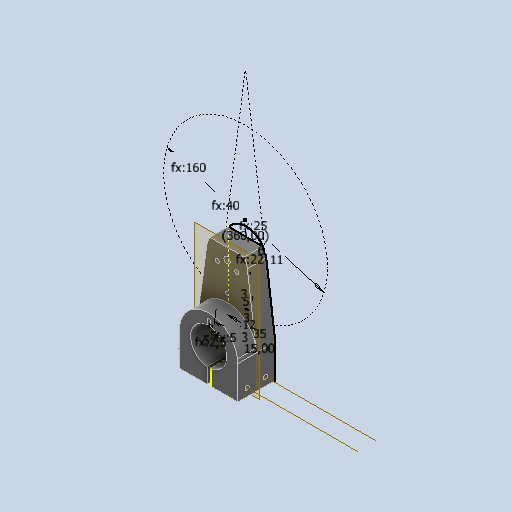
# Autodesk Inventor part: GC_Motor_Aussenscheibe
Saved by Autodesk Inventor 2022 (Build 260153000, 153)
## iProperties
Created: 2022-08-03
Part Number: GC_Motor_Aussenscheibe
Material: PBT-Kunststoff
Document SubType Name: Modeling
Designer: alexw
Mass: 147.379 g
Surface Area: 260.819 cm^2
Volume: 112.503 cm^3
Density: 1.31 g/cm^3
Appearance: Glatt - Schwarz
Author: alexw
Autodesk Inventor part; units mm, degrees
ref_plane "YZ Plane" through (0, 0, 0) normal (1, 0, 0) x (0, 1, 0)
ref_plane "XZ Plane" through (0, 0, 0) normal (0, 1, 0) x (-1, 0, 0)
ref_plane "XY Plane" through (0, 0, 0) normal (0, 0, 1) x (1, 0, 0)
sketch "Skizze1" plane through (0, 0, 0) normal (0, 0, 1) x (1, 0, 0)
  circle A0 centre (0, 0) radius 20 construction
  line L0 (-19.8289, 2.6105) -> (-28.5983, -64)
  line L1 (19.8289, 2.6105) -> (28.5983, -64)
  circle A1 centre (0, 0) radius 11 construction
  line L2 (0, 0) -> (0, 20) construction
  line L3 (0, 0) -> (0, -96.5) construction
  circle A2 centre (0, -64) radius 17.5
  line L4 (-19.8289, 2.6105) -> (0, 153.226) construction
  line L5 (19.8289, 2.6105) -> (0, 153.226) construction
  circle A3 centre (0, 25) radius 80 construction
  circle A4 centre (0, -64) radius 6 construction
  arc A5 (19.8289, 2.6105) -> (-19.8289, 2.6105) centre (0, 0) ccw
  line L6 (28.5983, -64) -> (28.5983, -96.5)
  line L7 (28.5983, -96.5) -> (-28.5983, -96.5)
  line L8 (-28.5983, -96.5) -> (-28.5983, -64)
  line L9 (0, -64) -> (-28.5983, -64) construction
  line L10 (0, -89) -> (-28.5983, -89) construction
  line L11 (0, -86.5) -> (-28.5983, -86.5) construction
  line L12 (0, -91.5) -> (-28.5983, -91.5) construction
  line L13 (1.5, -64) -> (-1.5, -64)
  line L14 (-1.5, -64) -> (-1.5, -96.5)
  line L15 (-1.5, -96.5) -> (1.5, -96.5)
  line L16 (1.5, -96.5) -> (1.5, -64)
  line L17 (-16.7033, 11) -> (16.7033, 11)
  circle A6 centre (0, 0) radius 3
  line L18 (-1.5, -46.5644) -> (-1.5, -41.5644)
  arc A7 (1.5, -41.5644) -> (-1.5, -41.5644) centre (0, -41.5644) ccw
  line L19 (1.5, -41.5644) -> (1.5, -46.5644)
  line L20 (1.5, -46.5644) -> (-1.5, -46.5644)
  point P0 (0, 11)
  point P1 (-9.5263, -5.5)
  point P2 (9.5263, -5.5)
  point P3 (0, -55)
  point P4 (0, -58)
  point P5 (0, -46.5)
  point P6 (0, -81.5)
  point P7 (-1.5, -81.4356)
  point P8 (1.5, -81.4356)
  point P9 (0, -46.5644)
  dimension "d9" = 22
  dimension "d54" = 160
  dimension "d56" = 12
  dimension "d2" = 360
  dimension "d10" = 40
  dimension "d47" = 25
  dimension "d51" = 3
  dimension "d52" = 15
  dimension "d55" = 35
  dimension "d61" = 5
  dimension "d62" = 2.5
  dimension "d63" = 5
  dimension "d65" = 3
  dimension "d66" = 5
  dimension "d81" = 11
  dimension "d82" = 6
  dimension "d85" = 3
  dimension "d86" = 5
  constraints: 40 end point, 13 point on circle, 7 perpendicular, 6 point on line, 6 tangent, 5 centre point, 5 coincident, 3 collinear, 3 horizontal, 3 midpoint, 3 parallel, 3 vertical, 3 vertical alignment, 1 equal length, 22 other
  measures "d10" diameter of A0
  measures "d47" distance of point (0, 25) point (0, 0)
  measures "d51" distance of point (0, -58) point (0, -55)
  measures "d52" angle of L1 L0
  measures "d55" diameter of A2
  measures "d61" distance between parallel lines of L11 L12
  measures "d62" distance between parallel lines of L12 L10
  measures "d63" distance between parallel lines of L12 L7
  measures "d65" distance between parallel lines of L14 L16
  measures "d66" distance from line of L11 A2.end
  measures "d81" distance from line of L17 point (0, 0)
  measures "d82" diameter of A6
  measures "d85" distance between parallel lines of L18 L19
  measures "d86" distance from line of A7.centre L20
extrude "Extrusion1" add sketch "Skizze1" along normal blind 18 contours A5 L17 L1 L6 L7 L16 A2 L19 A7 L18 L14 L8 L0
hole "Bohrung1" at (-9.5263, -5.5, 0) at (9.5263, -5.5, 0) direction (0, 0, 1) diameter 4 end through all
sketch "Skizze4" plane through (0, 0, 18) normal (0, 0, 1) x (1, 0, 0)
  circle A0 centre (0, -64) radius 28.3537
  line L0 (28.5983, -64) -> (19.8289, 2.6105) projected
  line L1 (-28.5983, -64) -> (-28.5983, -96.5) projected
  line L2 (-19.8289, 2.6105) -> (-28.5983, -64) projected
  line L3 (28.5983, -96.5) -> (28.5983, -64) projected
  line L4 (1.5, -96.5) -> (28.5983, -96.5) projected
  line L5 (-28.5983, -96.5) -> (-1.5, -96.5) projected
  line L6 (-1.5, -96.5) -> (-1.5, -81.4356) projected
  arc A1 (1.5, -81.4356) -> (-1.5, -81.4356) centre (0, -64) ccw projected
  line L7 (1.5, -81.4356) -> (1.5, -96.5) projected
  line L8 (1.5, -96.5) -> (1.5, -81.4356)
  line L9 (-1.5, -46.5644) -> (-1.5, -41.5644) projected
  arc A2 (1.5, -41.5644) -> (-1.5, -41.5644) centre (0, -41.5644) ccw projected
  line L10 (1.5, -41.5644) -> (1.5, -46.5644) projected
  line L11 (1.5, -46.5644) -> (-1.5, -46.5644) projected
  point P0 (0, 0)
  point P1 (28.1111, -60.2991)
  point P2 (-28.1111, -60.2991)
  constraints: 2 end point, 1 centre point, 1 coincident, 1 tangent, 1 vertical
extrude "Extrusion2" add sketch "Skizze4" along normal blind 18 contours A0 L7 A1 L10 A2 L9 L6 | A0 L0 L3 L4 L7 | A0 L6 L5 L1 L2
ref_plane "Arbeitsebene1" through (0, 0, 18) normal (0, 0, 1) x (1, 0, 0)
sketch "Skizze2" plane through (1.5, -96.5, 0) normal (-1, 0, 0) x (0, 0, 1)
  line L0 (0, 15.0644) -> (0, 0) construction
  line L1 (0, 0) -> (36, 0) construction
  line L2 (0, 15.0644) -> (36, 15.0644) construction
  line L3 (0, 0) -> (18, 0) construction
  line L4 (0, 15.0644) -> (18, 0) construction
  line L5 (18, 15.0644) -> (0, 0) construction
  line L6 (36, 15.0644) -> (36, 0) projected
  line L7 (18, 129) -> (18, -21.5) construction
  point P0 (0, 96.5)
  point P1 (9, 7.5322)
  point P2 (27, 7.5322)
  constraints: 4 end point, 2 midpoint, 1 symmetric about line
hole "Bohrung3" at (1.5, -88.9678, 9) at (1.5, -88.9678, 27) direction (1, 0, 0) diameter 4.134 end through all thread size "M5x0.8" class "6H" standard "ISO Metric profile"
sketch "Skizze3" plane through (-28.5983, -96.5, 0) normal (-1, 0, 0) x (0, 0, 1)
  point P0 (0, 96.5)
  point P1 (9, 7.5322)
  point P2 (27, 7.5322)
hole "Bohrung4" at (-28.5983, -88.9678, 9) at (-28.5983, -88.9678, 27) direction (1, 0, 0) diameter 5.5 depth 27.0983 tip angle 118 counterbore diameter 10 counterbore depth 5.5 clearance for "Inbusschraube DIN EN ISO 4762" size "M5" standard "DIN"
sketch "Skizze5" plane through (1.5, -96.5, 0) normal (0, -1, 0) x (1, 0, 0)
  line L0 (38.5377, 27) -> (-41.5377, 27) construction
  line L1 (38.5377, 9) -> (-41.5377, 9) construction
  line L2 (-41.5377, 18) -> (38.5377, 18) construction
  line L3 (-3, 36) -> (0, 36) construction
  line L4 (-1.5, 36) -> (-1.5, 0) construction
  point P0 (13.5, 18)
  point P1 (-16.5, 18)
  dimension "d87" = 15
  dimension "d88" = 30
  constraints: 2 end point, 2 point on line, 1 midpoint, 1 vertical
  measures "d87" distance from line of point (13.5, 18) L4
  measures "d88" distance of point (13.5, 18) point (-16.5, 18)
hole "Bohrung5" at (15, -96.5, 18) at (-15, -96.5, 18) direction (0, 1, 0) diameter 3.242 depth 11.8 tip angle 118 thread size "M4x0.7" class "6H" standard "ISO Metric profile"
sketch "Skizze6" plane through (0, 0, 0) normal (0, 0, -1) x (-1, 0, 0)
  arc A0 (28.1111, -60.2991) -> (-28.1111, -60.2991) centre (0, -64) ccw construction
  line L0 (0, 0) -> (0, -96.5) construction
  circle A1 centre (0, 0) radius 20 construction
  point P0 (0, -27.8963)
  point P1 (0, -20)
  point P2 (0, -35.6463)
  dimension "d96" = 15.6463
  dimension "d97" = 7.75
  constraints: 3 point on line, 1 point on circle, 1 vertical alignment, 1 other
  measures "d96" distance of point (0, -20) point (0, -35.646)
  measures "d97" distance of point (0, -27.896) point (0, -35.646)
hole "Bohrung6" at (0, -27.8963, 0) direction (0, 0, 1) diameter 3.242 end through all thread size "M4x0.7" class "6H" standard "ISO Metric profile"
equation "\"d9\" = FixationHole_Dia"
equation "\"d10\" = MotrGC_Part_OuterDia"
equation "\"d47\" = SmallCapston_Offset"
equation "\"FixationHole_Dia\" = 22"
equation "\"MotrGC_Part_OuterDia\" = 40"
equation "\"SmallCapston_Offset\" = 25"
